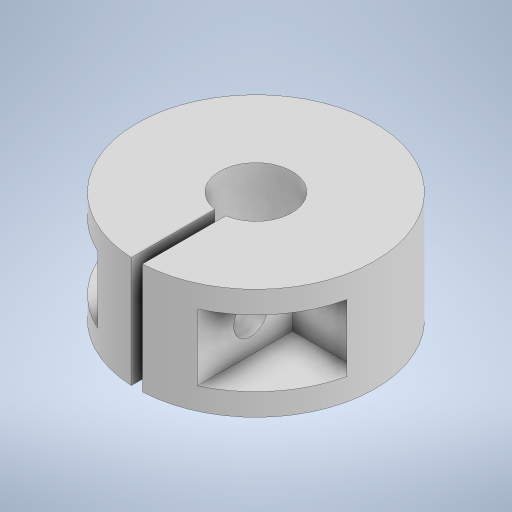
# Autodesk Inventor part: Motor Gear Connector
Saved by Autodesk Inventor 2023 (Build 270158000, 158)
## iProperties
Created: 2023-05-02
Part Number: Motor Gear Connector
Material: Generic
Document SubType Name: Modeling
Designer: mihal
Density: 1 g/cm^3
Appearance: Default
Author: mihal
Autodesk Inventor part; units mm, degrees
ref_plane "YZ Plane" through (0, 0, 0) normal (1, 0, 0) x (0, 1, 0)
sketch "Sketch1" plane through (0, 0, 0) normal (0, 1, 0) x (-1, 0, 0)
  circle A0 centre (0, 0) radius 3.25
  circle A1 centre (0, 0) radius 10.75
  dimension "d0" = 6.5
  dimension "d1" = 21.5
  constraints: 2 centre point, 2 coincident
  measures "d0" diameter of A0
  measures "d1" diameter of A1
extrude "Extrusion1" add sketch "Sketch1" along normal blind 10
sketch "Sketch2" plane through (0, 10, 0) normal (0, 1, 0) x (1, 0, 0)
  circle A0 centre (0, 0) radius 10.75 projected
  circle A1 centre (0, 0) radius 3.25 projected
  circle A2 centre (0, 0) radius 3.25 projected
  line L0 (-0.5, -3.2113) -> (-0.5, -10.7384)
  circle A3 centre (0, 0) radius 10.75 projected
  line L1 (0.5, -3.2113) -> (0.5, -10.7384)
  line L2 (0, -3.25) -> (0, -10.75) construction
  point P0 (0.5, -3.2113)
  dimension "d5" = 0.5
  dimension "d6" = 0.5
  constraints: 6 end point, 6 point on circle, 4 vertical
  measures "d5" distance between parallel lines of L1 L2
  measures "d6" distance between parallel lines of L2 L0
extrude "Extrusion2" cut sketch "Sketch2" against normal blind 10 contours L0 A1 L1 A0 picked at (-0.0556, -5.7467)
ref_plane "Work Plane1" through (10.5, 10, 3.2113) normal (-1, 0, 0) x (0, 0, 1)
sketch "Sketch3" plane through (10.5, 10, 3.2113) normal (-1, 0, 0) x (0, 0, 1)
  line L0 (0, -10) -> (0, 0) projected
  line L1 (7.5271, 0) -> (7.5271, -10) projected
  line L2 (0, -5) -> (7.5271, -5)
  line L3 (7.5271, -5) -> (7.5271, -2)
  line L4 (7.5271, -2) -> (0, -2)
  line L5 (0, -2) -> (0, -5)
  line L6 (0, -5) -> (7.5271, -5)
  line L7 (7.5271, -5) -> (7.5271, -8)
  line L8 (7.5271, -8) -> (0, -8)
  line L9 (0, -8) -> (0, -5)
  line L10 (0, -8) -> (-2, -8)
  line L11 (-2, -8) -> (-2, -2)
  line L12 (-2, -2) -> (0, -2)
  line L13 (0, -2) -> (0, -8)
  point P0 (-3.2113, -10)
  dimension "d10" = 3
  dimension "d11" = 3
  dimension "d20" = 2
  constraints: 24 end point, 6 parallel, 3 horizontal, 3 perpendicular, 2 point on line, 1 midpoint
  measures "d10" distance of L3.end L2.end
  measures "d11" distance of L6.end L7.end
  measures "d20" distance of L11.end L12.end
extrude "Extrusion3" cut sketch "Sketch3" along normal blind 6
ref_plane "Work Plane2" through (-10.5, 10, 10.7384) normal (1, 0, 0) x (0, 0, -1)
sketch "Sketch4" plane through (-10.5, 10, 10.7384) normal (1, 0, 0) x (0, 0, -1)
  line L0 (0, 0) -> (0, -10) projected
  line L1 (7.5271, -10) -> (7.5271, 0) projected
  line L2 (0, -5) -> (7.5271, -5)
  line L3 (7.5271, -5) -> (7.5271, -2)
  line L4 (7.5271, -2) -> (0, -2)
  line L5 (0, -2) -> (0, -5)
  line L6 (0, -5) -> (7.5271, -5)
  line L7 (7.5271, -5) -> (7.5271, -8)
  line L8 (7.5271, -8) -> (0, -8)
  line L9 (0, -8) -> (0, -5)
  line L10 (7.5271, -2) -> (9.5271, -2)
  line L11 (9.5271, -2) -> (9.5271, -8)
  line L12 (9.5271, -8) -> (7.5271, -8)
  line L13 (7.5271, -8) -> (7.5271, -2)
  point P0 (10.7384, -10)
  dimension "d15" = 3
  dimension "d16" = 3
  dimension "d21" = 2
  constraints: 24 end point, 6 parallel, 3 horizontal, 3 perpendicular, 2 point on line, 1 midpoint
  measures "d15" distance of L3.end L2.end
  measures "d16" distance of L6.end L7.end
  measures "d21" distance of L11.end L12.end
extrude "Extrusion4" cut sketch "Sketch4" along normal blind 6
sketch "Sketch5" plane through (4.5, 10, 3.2113) normal (1, 0, 0) x (0, 0, -1)
  line L0 (-6.5515, -8) -> (-6.5515, -2) projected
  line L1 (-6.5515, -2) -> (2, -2) projected
  circle A0 centre (-1.7581, -5) radius 1.55
  line L2 (2, -8) -> (-6.5515, -8) projected
  line L3 (2, -2) -> (-6.5515, -2) projected
  line L4 (-2.7084, -2) -> (-2.7084, -8) construction
  line L5 (-6.5515, -8) -> (2, -8) projected
  line L6 (1.1347, -8) -> (1.1347, -2) projected
  line L7 (1.1347, -5) -> (-6.5515, -5) construction
  line L8 (-6.5515, -2) -> (-6.5515, -8) projected
  line L9 (2, -2) -> (2, -8) projected
  point P0 (3.2113, -10)
  dimension "d19" = 3.1
  constraints: 4 end point, 2 midpoint, 2 point on line, 1 centre point
  measures "d19" diameter of A0
extrude "Extrusion5" cut sketch "Sketch5" against normal blind 10 contours A0
body "Solid1"
